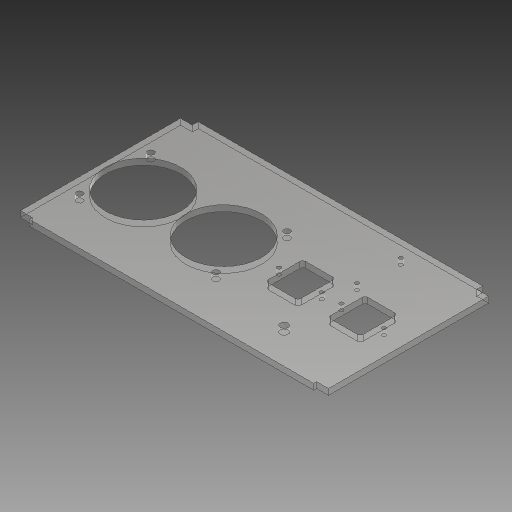
# Autodesk Inventor part: SeitenOben
Saved by Autodesk Inventor 2019 (Build 230136000, 136)
## iProperties
Created: 2018-04-27
Part Number: SeitenOben
Material: Polycarbonate, Clear
Document SubType Name: Modeling
Designer: Phil Erle
Density: 1.2 g/cm^3
Appearance: Polycarbonate - Clear
Author: Phil Erle
Autodesk Inventor part; units mm, degrees
ref_plane "YZ Plane" through (0, 0, 0) normal (1, 0, 0) x (0, 1, 0)
ref_plane "XZ Plane" through (0, 0, 0) normal (0, 1, 0) x (-1, 0, 0)
ref_plane "XY Plane" through (0, 0, 0) normal (0, 0, 1) x (1, 0, 0)
sketch "Sketch1" plane through (0, 0, 0) normal (0, 0, 1) x (1, 0, 0)
  line L0 (-130, 67.5) -> (-130, -67.5)
  line L1 (-130, -67.5) -> (-120, -67.5)
  line L2 (-120, -67.5) -> (-120, -70)
  line L3 (-120, -70) -> (120, -70)
  line L4 (120, -70) -> (120, -67.5)
  line L5 (120, -67.5) -> (130, -67.5)
  line L6 (130, -67.5) -> (130, 67.5)
  line L7 (130, 67.5) -> (120, 67.5)
  line L8 (120, 67.5) -> (120, 72.5)
  line L9 (120, 72.5) -> (-120, 72.5)
  line L10 (-120, 72.5) -> (-120, 67.5)
  line L11 (-130, 67.5) -> (-120, 67.5)
  point P0 (0, 0)
  point P1 (0, 72.5)
  point P2 (130, 0)
  point P3 (-130, 0)
  dimension "d0" = 5
  dimension "d1" = 240
  dimension "d2" = 10
  dimension "d3" = 10
  dimension "d4" = 2.5
  dimension "d5" = 135
  constraints: 24 end point, 8 perpendicular, 7 point on line, 3 midpoint, 1 horizontal alignment, 1 vertical, 1 vertical alignment
  measures "d0" distance of L7.end L8.end
  measures "d1" distance of L8.end L9.end
  measures "d2" distance of L0.start L10.end
  measures "d3" distance of L6.end L7.end
  measures "d4" distance of L3.end L4.end
  measures "d5" distance between parallel lines of L1 L11
extrude "Extrusion1" add sketch "Sketch1" along normal blind 5
sketch "Sketch2" plane through (0, 0, 5) normal (0, 0, 1) x (1, 0, 0)
  line L0 (25, -15.75) -> (52.5, -15.75)
  line L1 (52.5, -15.75) -> (52.5, 15.75)
  line L2 (52.5, 15.75) -> (25, 15.75)
  line L3 (25, 15.75) -> (25, -15.75)
  line L4 (77.5, -15.75) -> (105, -15.75)
  line L5 (105, -15.75) -> (105, 15.75)
  line L6 (105, 15.75) -> (77.5, 15.75)
  line L7 (77.5, 15.75) -> (77.5, -15.75)
  line L8 (130, -67.5) -> (130, 67.5) projected
  point P0 (0, 0)
  point P1 (25, 0)
  point P2 (77.5, 0)
  dimension "d8" = 27.5
  dimension "d9" = 31.5
  dimension "d10" = 27.5
  dimension "d11" = 31.5
  dimension "d12" = 130
  dimension "d13" = 25
  dimension "d14" = 25
  constraints: 16 end point, 4 parallel, 2 horizontal, 2 horizontal alignment, 2 midpoint, 2 perpendicular
  measures "d8" distance of L1.end L2.end
  measures "d9" distance of L2.end L0.start
  measures "d10" distance of L5.end L6.end
  measures "d11" distance of L6.end L4.start
  measures "d12" distance from line of L8 point (0, 0)
  measures "d13" distance from line of point (0, 0) L3
  measures "d14" distance between parallel lines of L1 L7
extrude "Extrusion2" cut sketch "Sketch2" against normal through all
sketch "Sketch3" plane through (0, 0, 5) normal (0, 0, 1) x (1, 0, 0)
  line L0 (20.75, 0) -> (56.75, 0) construction
  line L1 (25, 15.75) -> (52.5, 15.75) projected
  line L2 (77.5, 15.75) -> (105, 15.75) projected
  line L3 (73.25, 0) -> (109.25, 0) construction
  point P0 (0, 0)
  point P1 (38.75, 0)
  point P2 (38.75, 15.75)
  point P3 (91.25, 0)
  point P4 (91.25, 15.75)
  dimension "d17" = 36
  dimension "d18" = 36
  constraints: 4 coincident, 4 end point, 4 midpoint, 2 horizontal, 2 horizontal alignment, 2 vertical alignment
  measures "d17" distance of L0.start L0.end
  measures "d18" distance of L3.start L3.end
hole "Hole1" at (20.75, 0, 5) at (56.75, 0, 5) at (73.25, 0, 5) at (109.25, 0, 5) direction (0, 0, -1) diameter 3.4 depth 8 tip angle 118 clearance for "Countersunk Flat Head Screw DIN EN ISO 2009" size "M3" standard "DIN"
fillet "Fillet1" radius 2.5 8 edges at (25, 15.75, 2.5) (77.5, 15.75, 2.5) (105, 15.75, 2.5) (52.5, 15.75, 2.5) (52.5, -15.75, 2.5) (105, -15.75, 2.5) (25, -15.75, 2.5) (77.5, -15.75, 2.5)
sketch "Sketch5" plane through (0, 0, 5) normal (0, 0, 1) x (1, 0, 0)
  circle A0 centre (-94, 0) radius 32
  circle A1 centre (-26, 0) radius 32
  line L0 (-130, 67.5) -> (-130, -67.5) projected
  point P0 (0, 0)
  dimension "d34" = 64
  dimension "d35" = 68
  dimension "d36" = 36
  dimension "d37" = 64
  constraints: 2 centre point, 2 horizontal alignment
  measures "d34" diameter of A1
  measures "d35" distance of A1.centre A0.centre
  measures "d36" distance from line of A0.centre L0
  measures "d37" diameter of A0
extrude "Extrusion3" cut sketch "Sketch5" against normal through all
sketch "Sketch6" plane through (0, 0, 5) normal (0, 0, 1) x (1, 0, 0)
  point P0 (0, 0)
  point P1 (65, -40)
  dimension "d40" = 65
  dimension "d60" = 40
  measures "d40" horizontal distance of point (65, -40) point (0, 0)
  measures "d60" vertical distance of point (65, -40) point (0, 0)
hole "Hole3" at (65, -40, 5) direction (0, 0, -1) diameter 6.6 depth 8 tip angle 118 clearance for "Countersunk Flat Head Screw DIN EN ISO 2009" size "M6" standard "DIN"
sketch "Sketch7" plane through (0, 0, 5) normal (0, 0, 1) x (1, 0, 0)
  circle A0 centre (-94, 0) radius 32 construction
  circle A1 centre (-26, 0) radius 32 construction
  line L0 (-117.5, -30) -> (-2.5, -30) construction
  line L1 (-2.5, -30) -> (-2.5, 30) construction
  line L2 (-2.5, 30) -> (-117.5, 30) construction
  line L3 (-117.5, 30) -> (-117.5, -30) construction
  line L4 (-117.5, -30) -> (-2.5, 30) construction
  line L5 (-2.5, -30) -> (-117.5, 30) construction
  point P0 (0, 0)
  point P1 (-60, 0)
  point P2 (-60, 0)
  dimension "d49" = 68
  dimension "d50" = 34
  dimension "d51" = 115
  dimension "d52" = 60
  constraints: 12 end point, 4 coincident, 3 midpoint, 2 parallel, 1 horizontal, 1 horizontal alignment, 1 perpendicular
  measures "d49" distance of A1.centre A0.centre
  measures "d50" distance of point (-60, 0) A0.centre
  measures "d51" distance of L1.end L2.end
  measures "d52" distance of L0.end L1.end
hole "Hole4" at (-117.5, 30, 5) at (-117.5, -30, 5) at (-2.5, -30, 5) at (-2.5, 30, 5) direction (0, 0, -1) diameter 5.5 depth 8 tip angle 118 clearance for "Countersunk Flat Head Screw DIN EN ISO 2009" size "M5" standard "DIN"
sketch "Sketch8" plane through (0, 0, 5) normal (0, 0, 1) x (1, 0, 0)
  circle A0 centre (65, -40) radius 3.3 construction
  line L0 (65, 58.5) -> (65, 21.5) construction
  point P0 (0, 0)
  point P1 (65, 40)
  dimension "d62" = 37
  dimension "d63" = 40
  dimension "d71" = 0
  constraints: 2 coincident, 2 end point, 1 midpoint, 1 vertical
  measures "d62" distance of L0.start L0.end
  measures "d63" vertical distance of point (0, 0) point (65, 40)
  measures "d71" horizontal distance of A0.centre point (65, 40)
hole "Hole5" at (65, 21.5, 5) at (65, 58.5, 5) direction (0, 0, -1) diameter 3.4 depth 8 tip angle 118 clearance for "Countersunk Flat Head Screw DIN EN ISO 2009" size "M3" standard "DIN"
equation "\"d13\" = -0.666667 * d8 + 0.333333 * d12"
equation "\"d14\" = d13"
equation "\"d50\" = 0.5 * d49"
body "Solid1"
